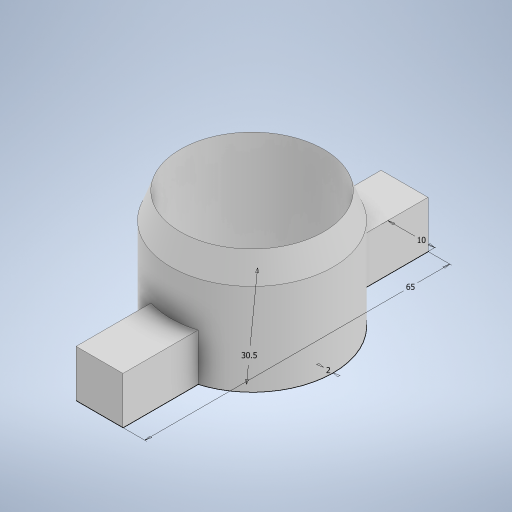
# Autodesk Inventor part: Pope8697-StopperCutter
Saved by Autodesk Inventor 2023 (Build 270158000, 158)
## iProperties
Created: 2024-07-12
Part Number: Pope8697-StopperCutter
Material: Generic
Document SubType Name: Modeling
Designer: incep
Density: 1 g/cm^3
Appearance: Default
Author: incep
## iProperties of the stored document Pope8697-StopperCutter_3DPrint.ipt
Created: 2024-07-12
Part Number: Pope8697-StopperCutter_3DPrint
Material: Generic
Document SubType Name: Modeling
Designer: incep
Density: 1 g/cm^3
Appearance: Default
Author: incep
Autodesk Inventor part; units mm, degrees
ref_plane "YZ Plane" through (0, 0, 0) normal (1, 0, 0) x (0, 1, 0)
ref_plane "XZ Plane" through (0, 0, 0) normal (0, 1, 0) x (-1, 0, 0)
ref_plane "XY Plane" through (0, 0, 0) normal (0, 0, 1) x (1, 0, 0)
sketch "Sketch1" plane through (0, 0, 0) normal (0, 1, 0) x (-1, 0, 0)
  circle A0 centre (0, 0) radius 15.25
  circle A1 centre (0, 0) radius 17.25
  line L0 (5, 32.5) -> (-5, 32.5)
  line L1 (-5, 32.5) -> (-5, -32.5)
  line L2 (-5, -32.5) -> (5, -32.5)
  line L3 (5, -32.5) -> (5, 32.5)
  point P0 (0, -32.5)
  point P1 (5, 0)
  point P2 (5, -16.5095)
  point P3 (-5, -16.5095)
  point P4 (-5, 16.5095)
  point P5 (5, 16.5095)
  dimension "d0" = 30.5
  dimension "d1" = 2
  dimension "d7" = 10
  dimension "d8" = 65
  constraints: 8 end point, 2 centre point, 2 midpoint, 2 parallel, 1 coincident, 1 horizontal, 1 horizontal alignment, 1 perpendicular, 1 vertical alignment
  measures "d0" diameter of A0
  measures "d1" radial gap between concentric circles of A0 A1
  measures "d7" distance of L1.end L2.end
  measures "d8" distance of L0.end L1.end
extrude "Extrusion1" add sketch "Sketch1" along normal blind 25 contours A0 L3 A1 | A0 L1 A1 L3 | L3 A1 L1 A0 | A0 L1 A1
chamfer "Chamfer1" distance 2 angle 70 1 edges at (17.25, 25, 0) measured on face at (-16.4162, 25, -1.3761)
extrude "Extrusion2" add sketch "Sketch1" along normal blind 10 contours A1 L1 L0 L3 | L3 L2 L1 A1
body "Solid1"
